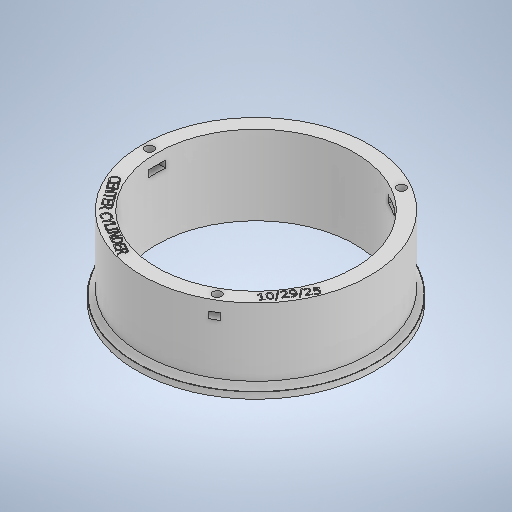
# Autodesk Inventor part: CenterCylinder_2
Saved by Autodesk Inventor 2025 (Build 290162000, 162)
## iProperties
Created: 2025-09-05
Part Number: CenterCylinder_2
Material: Generic
Document SubType Name: Modeling
Designer: mumin
Density: 1 g/cm^3
Appearance: Default
Author: mumin
Autodesk Inventor part; units mm, degrees
note: some values were not read from the file. Chosen so that the rebuilt part matches the saved one: direction of "Hole1".
ref_plane "YZ Plane" through (0, 0, 0) normal (1, 0, 0) x (0, 1, 0)
ref_plane "XZ Plane" through (0, 0, 0) normal (0, 1, 0) x (-1, 0, 0)
ref_plane "XY Plane" through (0, 0, 0) normal (0, 0, 1) x (1, 0, 0)
sketch "Sketch1" plane through (0, 0, 0) normal (0, 1, 0) x (-1, 0, 0)
  circle A0 centre (0, 0) radius 51
  circle A1 centre (0, 0) radius 47.55
  circle A2 centre (0, 0) radius 54.45
  dimension "d0" = 102
  dimension "d6" = 95.1
  dimension "d7" = 108.9
  constraints: 3 centre point, 2 coincident
  measures "d0" diameter of A0
  measures "d6" diameter of A1
  measures "d7" diameter of A2
extrude "Base" add sketch "Sketch1" along normal blind 30 contours A0 | A2
sketch "Sketch2" plane through (0, 30, 0) normal (0, 1, 0) x (1, 0, 0)
  line L0 (-51, 3.9837) -> (-47.55, 1.9919)
  line L1 (-47.55, 1.9919) -> (-47.55, -1.9919)
  line L2 (-47.55, -1.9919) -> (-51, -3.9837)
  line L3 (-51, -3.9837) -> (-54.45, -1.9919)
  line L4 (-54.45, -1.9919) -> (-54.45, 1.9919)
  line L5 (-54.45, 1.9919) -> (-51, 3.9837)
  circle A0 centre (0, 0) radius 54.45 projected
  circle A1 centre (0, 0) radius 47.55 projected
  line L6 (-51, -3.9837) -> (-47.2749, -3.9837)
  line L7 (-47.2749, -3.9837) -> (-47.2749, 3.9837)
  line L8 (-47.2749, 3.9837) -> (-51, 3.9837)
  line L9 (-51, 3.9837) -> (-51, -3.9837)
  point P0 (-51, 0)
  point P1 (-54.4128, 2.0134)
  point P2 (-54.4128, -2.0134)
  point P3 (-47.3828, -3.9837)
  point P4 (-47.55, 0)
  point P5 (-47.3828, 3.9837)
  constraints: 20 end point, 2 parallel, 2 tangent, 1 horizontal, 1 perpendicular, 13 other
extrude "Nut Seat" cut sketch "Sketch2" against normal blind 3.2 contours L8 A1 L1 L0 | L9 L3 A0 L5 | L0 L1 L2 L9 | L8 L7 L6 A1 | A1 L6 L7 L8 | L2 L1 A1 L6
pattern_circular "Circular Pattern1" count 3 over 360 about axis through (0, 0, 0) along (0, 1, 0) of "Nut Seat"
sketch "Sketch3" plane through (0, 30, 0) normal (0, 1, 0) x (1, 0, 0)
  circle A0 centre (0, 0) radius 47.55
  circle A1 centre (0, 0) radius 54.45
  constraints: 2 centre point, 2 coincident
extrude "Top Slice" add sketch "Sketch3" along normal blind 5
sketch "Sketch4" plane through (0, 35, 0) normal (0, 1, 0) x (1, 0, 0)
  line L0 (-76.23, 0) -> (76.23, 0) projected
  point P0 (0, 0)
  point P1 (-51, 0)
  dimension "d22" = 51
  constraints: 1 point on line
  measures "d22" distance of point (0, 0) point (-51, 0)
hole "Hole1" at (-51, 35, 0) direction (0, -1, 0) diameter 4.2 depth 5
pattern_circular "Circular Pattern2" count 3 over 360 about axis through (0, 0, 0) along (0, 1, 0) of "Hole1"
sketch "Sketch5" plane through (0, 0, 0) normal (0, -1, 0) x (1, 0, 0)
  circle A0 centre (0, 0) radius 47.55
  circle A1 centre (0, 0) radius 57.192
  constraints: 2 centre point, 2 coincident
extrude "Lip" add sketch "Sketch5" along normal blind 3
chamfer "Chamfer 1" distance 2.5 angle 45 1 edges at (54.45, 0, 0)
sketch "Sketch6" plane through (0, 35, 0) normal (0, 1, 0) x (1, 0, 0)
  line L0 (-45.9775, -18.336) -> (-33.9041, -35.5658) construction
  line L1 (-33.9041, -35.5658) -> (-37.9109, -38.3734) construction
  line L2 (-37.9109, -38.3734) -> (-49.9843, -21.1436) construction
  line L3 (-49.9843, -21.1436) -> (-45.9775, -18.336) construction
  line L4 (-34.2483, -35.5022) -> (-12.0289, -48.4135) construction
  line L5 (-12.0289, -48.4135) -> (-14.4649, -52.6058) construction
  line L6 (-14.4649, -52.6058) -> (-36.6844, -39.6946) construction
  line L7 (-36.6844, -39.6946) -> (-34.2483, -35.5022) construction
  line L8 (34.4629, -34.6295) -> (47.6298, -15.5928) construction
  line L9 (47.6298, -15.5928) -> (51.8853, -18.5361) construction
  line L10 (51.8853, -18.5361) -> (38.7184, -37.5728) construction
  line L11 (38.7184, -37.5728) -> (34.4629, -34.6295) construction
  spline S0 degree 2 poles (-48.241, -22.3247) (-48.4642, -22.0061) (-48.6268, -21.3165) (-48.5494, -20.9694) knots 0 0 0 1 2 2 2
  spline S1 degree 2 poles (-48.5494, -20.9694) (-48.4747, -20.6242) (-47.9883, -19.9627) (-47.5742, -19.6725) knots 0 0 0 1 2 2 2
  spline S2 degree 2 poles (-47.5742, -19.6725) (-47.1627, -19.3842) (-46.4052, -19.1661) (-46.04, -19.207) knots 0 0 0 1 2 2 2
  spline S3 degree 2 poles (-46.04, -19.207) (-45.682, -19.2491) (-45.0753, -19.6235) (-44.8428, -19.9553) knots 0 0 0 1 2 2 2
  spline S4 degree 2 poles (-44.8428, -19.9553) (-44.7275, -20.1199) (-44.5725, -20.4427) (-44.5241, -20.5909) knots 0 0 0 1 2 2 2
  spline S5 degree 2 poles (-44.5241, -20.5909) (-44.4842, -20.7213) (-44.428, -21.0104) (-44.4102, -21.1602) knots 0 0 0 1 2 2 2
  line L12 (-44.4102, -21.1602) -> (-44.9358, -21.5285)
  line L13 (-44.9358, -21.5285) -> (-44.96, -21.494)
  spline S6 degree 2 poles (-44.96, -21.494) (-44.9478, -21.3984) (-44.9256, -21.1137) (-44.9451, -20.9334) knots 0 0 0 1 2 2 2
  spline S7 degree 2 poles (-44.9451, -20.9334) (-44.9635, -20.7603) (-45.0824, -20.4042) (-45.2163, -20.2131) knots 0 0 0 1 2 2 2
  spline S8 degree 2 poles (-45.2163, -20.2131) (-45.3633, -20.0034) (-45.7981, -19.75) (-46.0613, -19.7246) knots 0 0 0 1 2 2 2
  spline S9 degree 2 poles (-46.0613, -19.7246) (-46.3253, -19.7038) (-46.9402, -19.9051) (-47.2561, -20.1265) knots 0 0 0 1 2 2 2
  spline S10 degree 2 poles (-47.2561, -20.1265) (-47.5932, -20.3627) (-47.9655, -20.865) (-48.0342, -21.1229) knots 0 0 0 1 2 2 2
  spline S11 degree 2 poles (-48.0342, -21.1229) (-48.0994, -21.3744) (-48.0054, -21.8588) (-47.8603, -22.0658) knots 0 0 0 1 2 2 2
  spline S12 degree 2 poles (-47.8603, -22.0658) (-47.7283, -22.2543) (-47.4103, -22.5104) (-47.2538, -22.5868) knots 0 0 0 1 2 2 2
  spline S13 degree 2 poles (-47.2538, -22.5868) (-47.1011, -22.6579) (-46.8331, -22.7353) (-46.7473, -22.7504) knots 0 0 0 1 2 2 2
  line L14 (-46.7473, -22.7504) -> (-46.725, -22.7823)
  line L15 (-46.725, -22.7823) -> (-47.2453, -23.1469)
  spline S14 degree 2 poles (-47.2453, -23.1469) (-47.372, -23.0734) (-47.5989, -22.9473) (-47.7362, -22.8417) knots 0 0 0 1 2 2 2
  spline S15 degree 2 poles (-47.7362, -22.8417) (-47.8844, -22.7318) (-48.1034, -22.5211) (-48.241, -22.3247) knots 0 0 0 1 2 2 2
  line L16 (-47.1837, -23.7093) -> (-43.9079, -21.4138)
  line L17 (-43.9079, -21.4138) -> (-42.4718, -23.4632)
  line L18 (-42.4718, -23.4632) -> (-42.8594, -23.7348)
  line L19 (-42.8594, -23.7348) -> (-43.9904, -22.1208)
  line L20 (-43.9904, -22.1208) -> (-44.8877, -22.7495)
  line L21 (-44.8877, -22.7495) -> (-43.8329, -24.2547)
  line L22 (-43.8329, -24.2547) -> (-44.2205, -24.5263)
  line L23 (-44.2205, -24.5263) -> (-45.2752, -23.0211)
  line L24 (-45.2752, -23.0211) -> (-46.4911, -23.873)
  line L25 (-46.4911, -23.873) -> (-45.3601, -25.4871)
  line L26 (-45.3601, -25.4871) -> (-45.7476, -25.7586)
  line L27 (-45.7476, -25.7586) -> (-47.1837, -23.7093)
  line L28 (-43.7703, -28.5805) -> (-44.1126, -28.0921)
  line L29 (-44.1126, -28.0921) -> (-42.3037, -24.6634)
  line L30 (-42.3037, -24.6634) -> (-45.1282, -26.6426)
  line L31 (-45.1282, -26.6426) -> (-45.4128, -26.2365)
  line L32 (-45.4128, -26.2365) -> (-42.137, -23.941)
  line L33 (-42.137, -23.941) -> (-41.7036, -24.5595)
  line L34 (-41.7036, -24.5595) -> (-43.3727, -27.6963)
  line L35 (-43.3727, -27.6963) -> (-40.7791, -25.8789)
  line L36 (-40.7791, -25.8789) -> (-40.4945, -26.2851)
  line L37 (-40.4945, -26.2851) -> (-43.7703, -28.5805)
  line L38 (-42.7695, -30.0087) -> (-39.8813, -27.9848)
  line L39 (-39.8813, -27.9848) -> (-40.6514, -26.8858)
  line L40 (-40.6514, -26.8858) -> (-40.2638, -26.6142)
  line L41 (-40.2638, -26.6142) -> (-38.4185, -29.2476)
  line L42 (-38.4185, -29.2476) -> (-38.8061, -29.5192)
  line L43 (-38.8061, -29.5192) -> (-39.5762, -28.4202)
  line L44 (-39.5762, -28.4202) -> (-42.4644, -30.4441)
  line L45 (-42.4644, -30.4441) -> (-42.7695, -30.0087)
  line L46 (-41.4618, -31.8749) -> (-38.186, -29.5794)
  line L47 (-38.186, -29.5794) -> (-36.75, -31.6288)
  line L48 (-36.75, -31.6288) -> (-37.1375, -31.9004)
  line L49 (-37.1375, -31.9004) -> (-38.2685, -30.2864)
  line L50 (-38.2685, -30.2864) -> (-39.1658, -30.9151)
  line L51 (-39.1658, -30.9151) -> (-38.1111, -32.4203)
  line L52 (-38.1111, -32.4203) -> (-38.4986, -32.6919)
  line L53 (-38.4986, -32.6919) -> (-39.5534, -31.1867)
  line L54 (-39.5534, -31.1867) -> (-40.7692, -32.0387)
  line L55 (-40.7692, -32.0387) -> (-39.6382, -33.6527)
  line L56 (-39.6382, -33.6527) -> (-40.0258, -33.9243)
  line L57 (-40.0258, -33.9243) -> (-41.4618, -31.8749)
  line L58 (-37.9145, -36.9373) -> (-38.3107, -36.3718)
  line L59 (-38.3107, -36.3718) -> (-37.7327, -34.4232)
  line L60 (-37.7327, -34.4232) -> (-38.0824, -33.9241)
  line L61 (-38.0824, -33.9241) -> (-39.3859, -34.8375)
  line L62 (-39.3859, -34.8375) -> (-39.6909, -34.4021)
  line L63 (-39.6909, -34.4021) -> (-36.4151, -32.1066)
  line L64 (-36.4151, -32.1066) -> (-35.8236, -32.9508)
  spline S16 degree 2 poles (-35.8236, -32.9508) (-35.6264, -33.2322) (-35.4215, -33.6546) (-35.4121, -33.9053) knots 0 0 0 1 2 2 2
  spline S17 degree 2 poles (-35.4121, -33.9053) (-35.4026, -34.156) (-35.6109, -34.5987) (-35.8684, -34.7792) knots 0 0 0 1 2 2 2
  spline S18 degree 2 poles (-35.8684, -34.7792) (-36.2268, -35.0303) (-36.9693, -35.0044) (-37.3056, -34.773) knots 0 0 0 1 2 2 2
  line L65 (-37.3056, -34.773) -> (-37.9145, -36.9373)
  spline S19 degree 2 poles (-36.221, -34.3494) (-36.0776, -34.249) (-35.928, -33.9937) (-35.9307, -33.8373) knots 0 0 0 1 2 2 2
  spline S20 degree 2 poles (-35.9307, -33.8373) (-35.9348, -33.7016) (-36.0573, -33.4194) (-36.1838, -33.2389) knots 0 0 0 1 2 2 2
  line L66 (-36.1838, -33.2389) -> (-36.487, -32.8062)
  line L67 (-36.487, -32.8062) -> (-37.7188, -33.6693)
  line L68 (-37.7188, -33.6693) -> (-37.4509, -34.0515)
  spline S21 degree 2 poles (-37.4509, -34.0515) (-37.3188, -34.24) (-37.0423, -34.4935) (-36.8662, -34.5245) knots 0 0 0 1 2 2 2
  spline S22 degree 2 poles (-36.8662, -34.5245) (-36.709, -34.5568) (-36.3909, -34.4685) (-36.221, -34.3494) knots 0 0 0 1 2 2 2
  spline S23 degree 2 poles (-34.6284, -40.0726) (-34.9648, -39.8771) (-35.4018, -39.3195) (-35.4773, -38.972) knots 0 0 0 1 2 2 2
  spline S24 degree 2 poles (-35.4773, -38.972) (-35.5544, -38.6273) (-35.3905, -37.8227) (-35.1365, -37.3855) knots 0 0 0 1 2 2 2
  spline S25 degree 2 poles (-35.1365, -37.3855) (-34.8841, -36.9511) (-34.2881, -36.4351) (-33.9394, -36.319) knots 0 0 0 1 2 2 2
  spline S26 degree 2 poles (-33.9394, -36.319) (-33.5969, -36.2069) (-32.889, -36.2921) (-32.5387, -36.4956) knots 0 0 0 1 2 2 2
  spline S27 degree 2 poles (-32.5387, -36.4956) (-32.3649, -36.5966) (-32.0888, -36.8246) (-31.9826, -36.9387) knots 0 0 0 1 2 2 2
  spline S28 degree 2 poles (-31.9826, -36.9387) (-31.8917, -37.0403) (-31.7193, -37.2792) (-31.6403, -37.4076) knots 0 0 0 1 2 2 2
  line L69 (-31.6403, -37.4076) -> (-31.9627, -37.9625)
  line L70 (-31.9627, -37.9625) -> (-31.9992, -37.9414)
  spline S29 degree 2 poles (-31.9992, -37.9414) (-32.0282, -37.8495) (-32.1276, -37.5818) (-32.221, -37.4263) knots 0 0 0 1 2 2 2
  spline S30 degree 2 poles (-32.221, -37.4263) (-32.3104, -37.2769) (-32.5677, -37.0036) (-32.7695, -36.8864) knots 0 0 0 1 2 2 2
  spline S31 degree 2 poles (-32.7695, -36.8864) (-32.9909, -36.7577) (-33.492, -36.7103) (-33.7415, -36.7977) knots 0 0 0 1 2 2 2
  spline S32 degree 2 poles (-33.7415, -36.7977) (-33.9898, -36.8896) (-34.4634, -37.3305) (-34.6572, -37.664) knots 0 0 0 1 2 2 2
  spline S33 degree 2 poles (-34.6572, -37.664) (-34.8641, -38.0199) (-34.9911, -38.6321) (-34.9452, -38.895) knots 0 0 0 1 2 2 2
  spline S34 degree 2 poles (-34.9452, -38.895) (-34.8988, -39.1507) (-34.6102, -39.5508) (-34.3916, -39.6778) knots 0 0 0 1 2 2 2
  spline S35 degree 2 poles (-34.3916, -39.6778) (-34.1926, -39.7935) (-33.7965, -39.8924) (-33.6224, -39.8961) knots 0 0 0 1 2 2 2
  spline S36 degree 2 poles (-33.6224, -39.8961) (-33.4539, -39.8965) (-33.1782, -39.8543) (-33.094, -39.832) knots 0 0 0 1 2 2 2
  line L71 (-33.094, -39.832) -> (-33.0604, -39.8515)
  line L72 (-33.0604, -39.8515) -> (-33.3796, -40.4009)
  spline S37 degree 2 poles (-33.3796, -40.4009) (-33.5254, -40.3873) (-33.7842, -40.3682) (-33.9532, -40.33) knots 0 0 0 1 2 2 2
  spline S38 degree 2 poles (-33.9532, -40.33) (-34.1339, -40.2925) (-34.421, -40.1931) (-34.6284, -40.0726) knots 0 0 0 1 2 2 2
  line L73 (-28.6564, -38.834) -> (-30.9456, -40.0832)
  line L74 (-30.9456, -40.0832) -> (-31.8348, -41.6134)
  line L75 (-31.8348, -41.6134) -> (-32.2944, -41.3463)
  line L76 (-32.2944, -41.3463) -> (-31.4329, -39.8637)
  line L77 (-31.4329, -39.8637) -> (-31.4535, -37.2087)
  line L78 (-31.4535, -37.2087) -> (-30.9434, -37.5051)
  line L79 (-30.9434, -37.5051) -> (-30.9336, -39.5465)
  line L80 (-30.9336, -39.5465) -> (-29.1441, -38.5507)
  line L81 (-29.1441, -38.5507) -> (-28.6564, -38.834)
  line L82 (-28.3426, -43.6426) -> (-30.3466, -42.4782)
  line L83 (-30.3466, -42.4782) -> (-28.3369, -39.0197)
  line L84 (-28.3369, -39.0197) -> (-27.8772, -39.2868)
  line L85 (-27.8772, -39.2868) -> (-29.6491, -42.3361)
  line L86 (-29.6491, -42.3361) -> (-28.1049, -43.2334)
  line L87 (-28.1049, -43.2334) -> (-28.3426, -43.6426)
  line L88 (-26.7759, -44.553) -> (-28.1156, -43.7746)
  line L89 (-28.1156, -43.7746) -> (-27.9104, -43.4214)
  line L90 (-27.9104, -43.4214) -> (-27.4704, -43.6771)
  line L91 (-27.4704, -43.6771) -> (-25.8711, -40.9249)
  line L92 (-25.8711, -40.9249) -> (-26.3112, -40.6692)
  line L93 (-26.3112, -40.6692) -> (-26.106, -40.3161)
  line L94 (-26.106, -40.3161) -> (-24.7663, -41.0945)
  line L95 (-24.7663, -41.0945) -> (-24.9715, -41.4476)
  line L96 (-24.9715, -41.4476) -> (-25.4115, -41.192)
  line L97 (-25.4115, -41.192) -> (-27.0108, -43.9442)
  line L98 (-27.0108, -43.9442) -> (-26.5707, -44.1999)
  line L99 (-26.5707, -44.1999) -> (-26.7759, -44.553)
  line L100 (-23.7322, -46.3217) -> (-24.2479, -46.022)
  line L101 (-24.2479, -46.022) -> (-24.0454, -42.1507)
  line L102 (-24.0454, -42.1507) -> (-25.7782, -45.1328)
  line L103 (-25.7782, -45.1328) -> (-26.207, -44.8836)
  line L104 (-26.207, -44.8836) -> (-24.1973, -41.4251)
  line L105 (-24.1973, -41.4251) -> (-23.5443, -41.8046)
  line L106 (-23.5443, -41.8046) -> (-23.7425, -45.3522)
  line L107 (-23.7425, -45.3522) -> (-22.1514, -42.614)
  line L108 (-22.1514, -42.614) -> (-21.7226, -42.8631)
  line L109 (-21.7226, -42.8631) -> (-23.7322, -46.3217)
  spline S39 degree 2 poles (-19.3014, -46.587) (-19.5766, -47.0606) (-20.4035, -47.5998) (-20.8496, -47.6255) knots 0 0 0 1 2 2 2
  spline S40 degree 2 poles (-20.8496, -47.6255) (-21.2091, -47.6378) (-21.8152, -47.4356) (-22.2356, -47.1913) knots 0 0 0 1 2 2 2
  line L110 (-22.2356, -47.1913) -> (-23.0316, -46.7288)
  line L111 (-23.0316, -46.7288) -> (-21.0219, -43.2703)
  line L112 (-21.0219, -43.2703) -> (-20.2343, -43.7279)
  spline S41 degree 2 poles (-20.2343, -43.7279) (-19.7467, -44.0113) (-19.2764, -44.4795) (-19.1552, -44.7224) knots 0 0 0 1 2 2 2
  spline S42 degree 2 poles (-19.1552, -44.7224) (-18.9503, -45.1376) (-19.0082, -46.0825) (-19.3014, -46.587) knots 0 0 0 1 2 2 2
  spline S43 degree 2 poles (-19.7774, -46.3029) (-19.5461, -45.9049) (-19.4822, -45.1885) (-19.65, -44.8772) knots 0 0 0 1 2 2 2
  spline S44 degree 2 poles (-19.65, -44.8772) (-19.7715, -44.6605) (-20.1321, -44.3197) (-20.4432, -44.1389) knots 0 0 0 1 2 2 2
  line L113 (-20.4432, -44.1389) -> (-20.7935, -43.9354)
  line L114 (-20.7935, -43.9354) -> (-22.3407, -46.5979)
  line L115 (-22.3407, -46.5979) -> (-21.9903, -46.8015)
  spline S45 degree 2 poles (-21.9903, -46.8015) (-21.6848, -46.979) (-21.1654, -47.1496) (-20.9011, -47.127) knots 0 0 0 1 2 2 2
  spline S46 degree 2 poles (-20.9011, -47.127) (-20.5656, -47.1045) (-20.0119, -46.7064) (-19.7774, -46.3029) knots 0 0 0 1 2 2 2
  line L116 (-19.8057, -48.6033) -> (-17.796, -45.1448)
  line L117 (-17.796, -45.1448) -> (-15.6324, -46.402)
  line L118 (-15.6324, -46.402) -> (-15.8701, -46.8112)
  line L119 (-15.8701, -46.8112) -> (-17.5742, -45.8211)
  line L120 (-17.5742, -45.8211) -> (-18.1246, -46.7684)
  line L121 (-18.1246, -46.7684) -> (-16.5355, -47.6918)
  line L122 (-16.5355, -47.6918) -> (-16.7733, -48.101)
  line L123 (-16.7733, -48.101) -> (-18.3624, -47.1776)
  line L124 (-18.3624, -47.1776) -> (-19.1083, -48.4612)
  line L125 (-19.1083, -48.4612) -> (-17.4042, -49.4514)
  line L126 (-17.4042, -49.4514) -> (-17.642, -49.8606)
  line L127 (-17.642, -49.8606) -> (-19.8057, -48.6033)
  line L128 (-14.461, -51.709) -> (-15.058, -51.3621)
  line L129 (-15.058, -51.3621) -> (-15.3514, -49.3508)
  line L130 (-15.3514, -49.3508) -> (-15.8783, -49.0447)
  line L131 (-15.8783, -49.0447) -> (-16.6779, -50.4208)
  line L132 (-16.6779, -50.4208) -> (-17.1375, -50.1537)
  line L133 (-17.1375, -50.1537) -> (-15.1279, -46.6952)
  line L134 (-15.1279, -46.6952) -> (-14.2366, -47.2131)
  spline S47 degree 2 poles (-14.2366, -47.2131) (-13.9395, -47.3857) (-13.5762, -47.6831) (-13.4624, -47.9066) knots 0 0 0 1 2 2 2
  spline S48 degree 2 poles (-13.4624, -47.9066) (-13.3487, -48.1302) (-13.3518, -48.6195) (-13.5098, -48.8914) knots 0 0 0 1 2 2 2
  spline S49 degree 2 poles (-13.5098, -48.8914) (-13.7296, -49.2697) (-14.4144, -49.5579) (-14.8168, -49.489) knots 0 0 0 1 2 2 2
  line L135 (-14.8168, -49.489) -> (-14.461, -51.709)
  spline S50 degree 2 poles (-14.0102, -48.6493) (-13.9223, -48.498) (-13.8936, -48.2034) (-13.9617, -48.0626) knots 0 0 0 1 2 2 2
  spline S51 degree 2 poles (-13.9617, -48.0626) (-14.0224, -47.9412) (-14.2521, -47.7365) (-14.4427, -47.6257) knots 0 0 0 1 2 2 2
  line L136 (-14.4427, -47.6257) -> (-14.8995, -47.3603)
  line L137 (-14.8995, -47.3603) -> (-15.6552, -48.6607)
  line L138 (-15.6552, -48.6607) -> (-15.2516, -48.8952)
  spline S52 degree 2 poles (-15.2516, -48.8952) (-15.0526, -49.0108) (-14.6952, -49.1248) (-14.5223, -49.079) knots 0 0 0 1 2 2 2
  spline S53 degree 2 poles (-14.5223, -49.079) (-14.3661, -49.0424) (-14.1144, -48.8287) (-14.0102, -48.6493) knots 0 0 0 1 2 2 2
  line L139 (39.3542, -34.9029) -> (38.2442, -36.5078)
  line L140 (38.2442, -36.5078) -> (37.9082, -36.2754)
  line L141 (37.9082, -36.2754) -> (38.3213, -35.6783)
  line L142 (38.3213, -35.6783) -> (36.1166, -34.1533)
  line L143 (36.1166, -34.1533) -> (35.7035, -34.7505)
  line L144 (35.7035, -34.7505) -> (35.4023, -34.5421)
  spline S54 degree 2 poles (35.4023, -34.5421) (35.6364, -34.2036) (35.6658, -33.7509) (35.4139, -33.5452) knots 0 0 0 1 2 2 2
  line L145 (35.4139, -33.5452) -> (35.6499, -33.2039)
  line L146 (35.6499, -33.2039) -> (38.6145, -35.2544)
  line L147 (38.6145, -35.2544) -> (39.0183, -34.6705)
  line L148 (39.0183, -34.6705) -> (39.3542, -34.9029)
  spline S55 degree 2 poles (39.544, -31.1126) (40.4291, -31.7247) (40.9023, -32.8127) (40.5317, -33.3486) knots 0 0 0 1 2 2 2
  spline S56 degree 2 poles (40.5317, -33.3486) (40.1555, -33.8924) (38.9583, -33.8171) (38.0918, -33.2178) knots 0 0 0 1 2 2 2
  spline S57 degree 2 poles (38.0918, -33.2178) (37.2014, -32.602) (36.7335, -31.5177) (37.106, -30.9791) knots 0 0 0 1 2 2 2
  spline S58 degree 2 poles (37.106, -30.9791) (37.4803, -30.438) (38.6856, -30.5188) (39.544, -31.1126) knots 0 0 0 1 2 2 2
  spline S59 degree 2 poles (40.1555, -32.371) (40.0371, -32.1946) (39.5728, -31.7946) (39.2342, -31.5604) knots 0 0 0 1 2 2 2
  spline S60 degree 2 poles (39.2342, -31.5604) (38.8957, -31.3263) (38.3602, -31.0348) (38.1462, -30.9852) knots 0 0 0 1 2 2 2
  spline S61 degree 2 poles (38.1462, -30.9852) (37.9321, -30.9357) (37.5984, -31.0478) (37.4712, -31.2318) knots 0 0 0 1 2 2 2
  spline S62 degree 2 poles (37.4712, -31.2318) (37.344, -31.4157) (37.3532, -31.7728) (37.4785, -31.962) knots 0 0 0 1 2 2 2
  spline S63 degree 2 poles (37.4785, -31.962) (37.6004, -32.1448) (38.079, -32.5468) (38.4016, -32.7699) knots 0 0 0 1 2 2 2
  spline S64 degree 2 poles (38.4016, -32.7699) (38.7482, -33.0097) (39.2416, -33.2878) (39.4708, -33.3439) knots 0 0 0 1 2 2 2
  spline S65 degree 2 poles (39.4708, -33.3439) (39.6857, -33.3979) (40.0337, -33.2879) (40.1665, -33.096) knots 0 0 0 1 2 2 2
  spline S66 degree 2 poles (40.1665, -33.096) (40.2919, -32.9147) (40.2827, -32.5576) (40.1555, -32.371) knots 0 0 0 1 2 2 2
  line L149 (38.9898, -28.0846) -> (42.25, -32.2432)
  line L150 (42.25, -32.2432) -> (41.9919, -32.6165)
  line L151 (41.9919, -32.6165) -> (38.7279, -28.4632)
  line L152 (38.7279, -28.4632) -> (38.9898, -28.0846)
  line L153 (44.0802, -28.0701) -> (42.6769, -30.0988)
  line L154 (42.6769, -30.0988) -> (42.2104, -29.7762)
  spline S67 degree 2 poles (42.2104, -29.7762) (42.1563, -29.4156) (42.0443, -28.7627) (41.9681, -28.4341) knots 0 0 0 1 2 2 2
  spline S68 degree 2 poles (41.9681, -28.4341) (41.8149, -27.7724) (41.5089, -27.1548) (41.245, -26.9722) knots 0 0 0 1 2 2 2
  spline S69 degree 2 poles (41.245, -26.9722) (41.1064, -26.8764) (40.8394, -26.8178) (40.7193, -26.8491) knots 0 0 0 1 2 2 2
  spline S70 degree 2 poles (40.7193, -26.8491) (40.5992, -26.8803) (40.3924, -27.0368) (40.3076, -27.1594) knots 0 0 0 1 2 2 2
  spline S71 degree 2 poles (40.3076, -27.1594) (40.2264, -27.2767) (40.1191, -27.5572) (40.0889, -27.6979) knots 0 0 0 1 2 2 2
  spline S72 degree 2 poles (40.0889, -27.6979) (40.0616, -27.817) (40.0484, -28.064) (40.0489, -28.1432) knots 0 0 0 1 2 2 2
  line L155 (40.0489, -28.1432) -> (40.0323, -28.1672)
  line L156 (40.0323, -28.1672) -> (39.5631, -27.8426)
  spline S73 degree 2 poles (39.5631, -27.8426) (39.5905, -27.6606) (39.7973, -27.0824) (39.9485, -26.8638) knots 0 0 0 1 2 2 2
  spline S74 degree 2 poles (39.9485, -26.8638) (40.2675, -26.4025) (41.1149, -26.2201) (41.5308, -26.5078) knots 0 0 0 1 2 2 2
  spline S75 degree 2 poles (41.5308, -26.5078) (41.7254, -26.6424) (41.988, -26.958) (42.0713, -27.1338) knots 0 0 0 1 2 2 2
  spline S76 degree 2 poles (42.0713, -27.1338) (42.1599, -27.3134) (42.2821, -27.7408) (42.3295, -27.9628) knots 0 0 0 1 2 2 2
  spline S77 degree 2 poles (42.3295, -27.9628) (42.4123, -28.3275) (42.5453, -29.1723) (42.5815, -29.4219) knots 0 0 0 1 2 2 2
  line L157 (42.5815, -29.4219) -> (43.6989, -27.8064)
  line L158 (43.6989, -27.8064) -> (44.0802, -28.0701)
  spline S78 degree 2 poles (42.101, -26.1848) (41.8477, -26.0097) (41.5408, -25.553) (41.4884, -25.304) knots 0 0 0 1 2 2 2
  spline S79 degree 2 poles (41.4884, -25.304) (41.4359, -25.0666) (41.548, -24.5569) (41.6881, -24.3543) knots 0 0 0 1 2 2 2
  spline S80 degree 2 poles (41.6881, -24.3543) (41.8448, -24.1277) (42.2513, -23.8649) (42.4893, -23.8285) knots 0 0 0 1 2 2 2
  spline S81 degree 2 poles (42.4893, -23.8285) (42.7886, -23.7833) (43.5041, -24.0023) (43.9547, -24.3139) knots 0 0 0 1 2 2 2
  spline S82 degree 2 poles (43.9547, -24.3139) (44.3626, -24.596) (44.9658, -25.2852) (45.0849, -25.6316) knots 0 0 0 1 2 2 2
  spline S83 degree 2 poles (45.0849, -25.6316) (45.2099, -25.9979) (45.1104, -26.7174) (44.8411, -27.1066) knots 0 0 0 1 2 2 2
  spline S84 degree 2 poles (44.8411, -27.1066) (44.7803, -27.1946) (44.6233, -27.3816) (44.5377, -27.4485) knots 0 0 0 1 2 2 2
  line L159 (44.5377, -27.4485) -> (44.1138, -27.1553)
  line L160 (44.1138, -27.1553) -> (44.1285, -27.134)
  spline S85 degree 2 poles (44.1285, -27.134) (44.1993, -27.1001) (44.4175, -26.9042) (44.5005, -26.7843) knots 0 0 0 1 2 2 2
  spline S86 degree 2 poles (44.5005, -26.7843) (44.7992, -26.3524) (44.5698, -25.4646) (44.0659, -25.0648) knots 0 0 0 1 2 2 2
  spline S87 degree 2 poles (44.0659, -25.0648) (44.0642, -25.3238) (43.9522, -25.7193) (43.8213, -25.9086) knots 0 0 0 1 2 2 2
  spline S88 degree 2 poles (43.8213, -25.9086) (43.6959, -26.0898) (43.4076, -26.3358) (43.1878, -26.4084) knots 0 0 0 1 2 2 2
  spline S89 degree 2 poles (43.1878, -26.4084) (42.9302, -26.4904) (42.3916, -26.3858) (42.101, -26.1848) knots 0 0 0 1 2 2 2
  spline S90 degree 2 poles (43.5481, -24.6909) (43.2149, -24.4604) (42.7088, -24.2917) (42.5186, -24.3217) knots 0 0 0 1 2 2 2
  spline S91 degree 2 poles (42.5186, -24.3217) (42.3456, -24.3439) (42.1273, -24.4886) (42.0462, -24.6059) knots 0 0 0 1 2 2 2
  spline S92 degree 2 poles (42.0462, -24.6059) (41.8581, -24.8778) (42.0242, -25.4696) (42.3921, -25.7241) knots 0 0 0 1 2 2 2
  spline S93 degree 2 poles (42.3921, -25.7241) (42.6, -25.8679) (42.9431, -25.9475) (43.1202, -25.8966) knots 0 0 0 1 2 2 2
  spline S94 degree 2 poles (43.1202, -25.8966) (43.2485, -25.8592) (43.4395, -25.6799) (43.5243, -25.5573) knots 0 0 0 1 2 2 2
  spline S95 degree 2 poles (43.5243, -25.5573) (43.622, -25.416) (43.7483, -25.0225) (43.7505, -24.8427) knots 0 0 0 1 2 2 2
  spline S96 degree 2 poles (43.7505, -24.8427) (43.7204, -24.8179) (43.6148, -24.737) (43.5481, -24.6909) knots 0 0 0 1 2 2 2
  line L161 (43.6014, -21.4171) -> (46.8617, -25.5757)
  line L162 (46.8617, -25.5757) -> (46.6035, -25.9489)
  line L163 (46.6035, -25.9489) -> (43.3396, -21.7956)
  line L164 (43.3396, -21.7956) -> (43.6014, -21.4171)
  line L165 (48.6918, -21.4026) -> (47.2886, -23.4313)
  line L166 (47.2886, -23.4313) -> (46.822, -23.1086)
  spline S97 degree 2 poles (46.822, -23.1086) (46.768, -22.7481) (46.6559, -22.0951) (46.5797, -21.7666) knots 0 0 0 1 2 2 2
  spline S98 degree 2 poles (46.5797, -21.7666) (46.4265, -21.1048) (46.1206, -20.4873) (45.8566, -20.3047) knots 0 0 0 1 2 2 2
  spline S99 degree 2 poles (45.8566, -20.3047) (45.718, -20.2089) (45.4511, -20.1503) (45.3309, -20.1816) knots 0 0 0 1 2 2 2
  spline S100 degree 2 poles (45.3309, -20.1816) (45.2108, -20.2128) (45.004, -20.3693) (44.9192, -20.4919) knots 0 0 0 1 2 2 2
  spline S101 degree 2 poles (44.9192, -20.4919) (44.8381, -20.6092) (44.7308, -20.8897) (44.7005, -21.0304) knots 0 0 0 1 2 2 2
  spline S102 degree 2 poles (44.7005, -21.0304) (44.6733, -21.1495) (44.6601, -21.3965) (44.6605, -21.4757) knots 0 0 0 1 2 2 2
  line L167 (44.6605, -21.4757) -> (44.6439, -21.4997)
  line L168 (44.6439, -21.4997) -> (44.1747, -21.1751)
  spline S103 degree 2 poles (44.1747, -21.1751) (44.2021, -20.9931) (44.4089, -20.4148) (44.5601, -20.1962) knots 0 0 0 1 2 2 2
  spline S104 degree 2 poles (44.5601, -20.1962) (44.8791, -19.735) (45.7265, -19.5526) (46.1424, -19.8403) knots 0 0 0 1 2 2 2
  spline S105 degree 2 poles (46.1424, -19.8403) (46.337, -19.9749) (46.5996, -20.2905) (46.6829, -20.4663) knots 0 0 0 1 2 2 2
  spline S106 degree 2 poles (46.6829, -20.4663) (46.7716, -20.6459) (46.8937, -21.0733) (46.9412, -21.2953) knots 0 0 0 1 2 2 2
  spline S107 degree 2 poles (46.9412, -21.2953) (47.024, -21.66) (47.157, -22.5047) (47.1932, -22.7544) knots 0 0 0 1 2 2 2
  line L169 (47.1932, -22.7544) -> (48.3106, -21.1389)
  line L170 (48.3106, -21.1389) -> (48.6918, -21.4026)
  spline S108 degree 2 poles (49.3303, -18.2457) (49.5675, -18.4098) (49.8676, -18.8421) (49.921, -19.084) knots 0 0 0 1 2 2 2
  spline S109 degree 2 poles (49.921, -19.084) (49.9745, -19.3259) (49.8619, -19.8589) (49.6849, -20.1149) knots 0 0 0 1 2 2 2
  spline S110 degree 2 poles (49.6849, -20.1149) (49.5227, -20.3495) (49.1015, -20.7361) (48.9027, -20.8469) knots 0 0 0 1 2 2 2
  line L171 (48.9027, -20.8469) -> (48.4362, -20.5242)
  line L172 (48.4362, -20.5242) -> (48.4583, -20.4922)
  spline S111 degree 2 poles (48.4583, -20.4922) (48.5307, -20.4674) (48.7576, -20.3445) (48.8795, -20.2593) knots 0 0 0 1 2 2 2
  spline S112 degree 2 poles (48.8795, -20.2593) (49.0152, -20.16) (49.2152, -19.9791) (49.3092, -19.8432) knots 0 0 0 1 2 2 2
  spline S113 degree 2 poles (49.3092, -19.8432) (49.4014, -19.7099) (49.4788, -19.3929) (49.4375, -19.2303) knots 0 0 0 1 2 2 2
  spline S114 degree 2 poles (49.4375, -19.2303) (49.396, -19.0795) (49.1938, -18.8135) (49.0178, -18.6918) knots 0 0 0 1 2 2 2
  spline S115 degree 2 poles (49.0178, -18.6918) (48.8419, -18.5701) (48.5515, -18.5112) (48.4142, -18.5502) knots 0 0 0 1 2 2 2
  spline S116 degree 2 poles (48.4142, -18.5502) (48.267, -18.5863) (48.0059, -18.8156) (47.8898, -18.9836) knots 0 0 0 1 2 2 2
  spline S117 degree 2 poles (47.8898, -18.9836) (47.7644, -19.1649) (47.5714, -19.5635) (47.5198, -19.6894) knots 0 0 0 1 2 2 2
  line L173 (47.5198, -19.6894) -> (45.8243, -18.5167)
  line L174 (45.8243, -18.5167) -> (47.0726, -16.7118)
  line L175 (47.0726, -16.7118) -> (47.4592, -16.9792)
  line L176 (47.4592, -16.9792) -> (46.504, -18.3601)
  line L177 (46.504, -18.3601) -> (47.3811, -18.9668)
  spline S118 degree 2 poles (47.3811, -18.9668) (47.4258, -18.8794) (47.5247, -18.7193) (47.569, -18.6553) knots 0 0 0 1 2 2 2
  spline S119 degree 2 poles (47.569, -18.6553) (47.7442, -18.402) (48.0684, -18.11) (48.3016, -18.0348) knots 0 0 0 1 2 2 2
  spline S120 degree 2 poles (48.3016, -18.0348) (48.5367, -17.957) (49.0317, -18.0392) (49.3303, -18.2457) knots 0 0 0 1 2 2 2
  point P0 (0, 0)
  constraints: 6 other
emboss "Emboss1" sketch "Sketch6" operation cut depth 1 direction (0, -1, 0)
body "Solid1"
